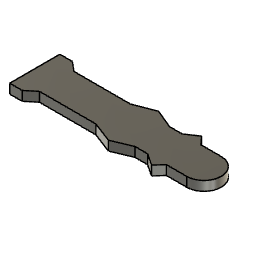
Watch Bands_ (Autodesk Fusion 360 design; units mm, degrees)
Autodesk Fusion 360 part; units mm, degrees
sketch "Sketch1" plane through (0, 0, 0) normal (0, 0, 1) x (1, 0, 0)
  line L0 (0, 0) -> (-119, 0)
  line L1 (-119, 0) -> (-119, 32)
  line L2 (-119, 32) -> (0, 32)
  line L3 (0, 32) -> (0, 0)
  line L4 (-105, 27.0131) -> (-111, 32)
  line L5 (-105, 27.0131) -> (-69, 27.0131)
  line L6 (-69, 27.0131) -> (-56, 32)
  line L7 (-105, 4.9869) -> (-69, 4.9869)
  line L8 (-105, 4.9869) -> (-111, 0)
  line L9 (-69, 4.9869) -> (-56, 0)
  line L10 (-44, 27) -> (-36, 27)
  line L11 (-44, 27) -> (-56, 32)
  line L12 (-36, 27) -> (-28.5, 32)
  line L13 (-28.5, 32) -> (-24, 27)
  line L14 (-24, 27) -> (0, 27)
  line L15 (-24, 5) -> (0, 5)
  line L16 (-28.5, 0) -> (-24, 5)
  line L17 (-36, 5) -> (-28.5, 0)
  line L18 (-44, 5) -> (-36, 5)
  line L19 (-44, 5) -> (-56, 0)
  circle A0 centre (-11, 16) radius 11
  dimension "d1" = 119
  dimension "d2" = 32
  dimension "d5" = 8
  dimension "d14" = 14
  dimension "d16" = 36
  dimension "d17" = 63
  dimension "d18" = 8
  dimension "d19" = 25
  dimension "d21" = 12
  constraint horizontal L0
  constraint vertical L1
  constraint horizontal L2
  constraint vertical L3
  constraint coincident L0.start L3.end
  constraint coincident L2 L4.end
  constraint horizontal L5
  constraint coincident L2 L6.end
  constraint horizontal L10
  constraint coincident L2 L12.end
  constraint coincident L3 L14.end
  constraint perpendicular L3 L14
  measures "d1" distance of L0.start L0.end
  measures "d2" distance of L0.start L2.end
  measures "d5" distance of L1.end L4.end
  measures "d14" distance of L1 L4.start
  measures "d16" distance of L4.start L5.end
  measures "d17" distance of L1 L6.end
  measures "d18" distance of L10.start L10.end
  measures "d19" horizontal distance of L5.end L10.start
  measures "d21" distance of L10.end L13.end
extrude "Extrude1" add sketch "Sketch1" along normal blind 6 contours L0 L1 L2 L4 L5 L6 L7 L8 L9 L10 L11 L12 L13 L14 L15 L16 L17 L18 L19 A0 | A0
equation "d16 = 50 mm - 14 mm"
